010 (Autodesk Fusion 360 design; units mm, degrees)
Autodesk Fusion 360 part; units mm, degrees
sketch "Esquisse1" plane through (0, 0, 0) normal (0, 0, 1) x (1, 0, 0)
  line L0 (-15, 10) -> (15, 10)
  line L1 (15, 10) -> (15, 0)
  line L2 (15, 0) -> (-15, 0)
  line L3 (-15, 0) -> (-15, 10)
  line L4 (0, 1.75) -> (0, 22.5)
  dimension "d1" = 30
  dimension "d2" = 10
  constraint horizontal L0
  constraint vertical L1
  constraint horizontal L2
  constraint vertical L3
  constraint coincident origin L2
  constraint symmetric L1 L3 L4
  measures "d1" distance of L0.start L0.end
  measures "d2" distance of L0.start L2.end
extrude "Extrusion1" add sketch "Esquisse1" along normal blind 46
sketch "Esquisse2" plane through (0, 0, 0) normal (0, 0, -1) x (1, 0, 0)
  line L0 (15, 0) -> (-15, 0)
  line L1 (-15, 0) -> (-15, -10)
  line L2 (-15, -10) -> (15, -10)
  line L3 (15, -10) -> (15, 0)
  point P0 (-11, -5)
  dimension "d5" = 11
  dimension "d6" = 5
  measures "d5" horizontal distance of origin P0
  measures "d6" distance of L0 P0
hole "Perçage1" at (-11, 5, 0) direction (0, 0, 1) diameter 2.5 depth 57 tip angle 118
mirror "Symétrie miroir1" about plane through (0, 0, 0) normal (1, 0, 0) of "Perçage1"
